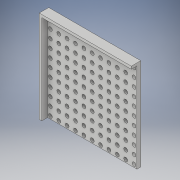
# Autodesk Inventor part: base
Saved by Autodesk Inventor 2018 (Build 220112000, 112)
## iProperties
Created: 2018-04-20
Part Number: base
Material: Generic
Document SubType Name: Modeling
Designer: 4070609
Density: 1 g/cm^3
Appearance: Default
Author: 4070609
Autodesk Inventor part; units mm, degrees
ref_plane "YZ Plane" through (0, 0, 0) normal (1, 0, 0) x (0, 1, 0)
ref_plane "XZ Plane" through (0, 0, 0) normal (0, 1, 0) x (-1, 0, 0)
ref_plane "XY Plane" through (0, 0, 0) normal (0, 0, 1) x (1, 0, 0)
sketch "Sketch1" plane through (0, 0, 0) normal (0, 0, 1) x (1, 0, 0)
  line L0 (0, 0) -> (48.4, 0)
  line L1 (48.4, 0) -> (48.4, 48.4)
  line L2 (48.4, 48.4) -> (0, 48.4)
  line L3 (0, 48.4) -> (0, 0)
  dimension "d0" = 48.4
  dimension "d1" = 48.4
  constraints: 8 end point, 2 parallel, 1 horizontal, 1 perpendicular
  measures "d0" distance of L2.end L1.end
  measures "d1" distance of L1.end L0.end
extrude "Extrusion1" add sketch "Sketch1" along normal blind 2
sketch "Sketch2" plane through (0, 0, 2) normal (0, 0, 1) x (1, 0, 0)
  line L0 (48.4, 0) -> (48.4, 48.4) projected
  line L1 (0, 48.4) -> (0, 0) projected
  line L2 (48.4, 48.4) -> (0, 48.4)
  line L3 (0, 48.4) -> (0, 47)
  line L4 (0, 47) -> (48.4, 47)
  line L5 (48.4, 47) -> (48.4, 48.4)
  line L6 (48.4, 48.4) -> (0, 48.4) projected
  line L7 (0, 0) -> (48.4, 0) projected
  line L8 (0, 48.4) -> (1.4, 48.4)
  line L9 (1.4, 48.4) -> (1.4, 0)
  line L10 (1.4, 0) -> (0, 0)
  line L11 (0, 0) -> (0, 48.4)
  dimension "d4" = 1.4
  dimension "d5" = 1.4
  constraints: 16 end point, 4 parallel, 2 horizontal, 2 perpendicular, 2 point on line
  measures "d4" distance of L3.end L2.end
  measures "d5" distance of L9.end L10.end
extrude "Extrusion2" add sketch "Sketch2" along normal blind 3 contours L4 L9 L2 L0 | L7 L1 L4 L9 | L4 L1 L2 L9
sketch "Sketch3" plane through (0, 0, 2) normal (0, 0, 1) x (1, 0, 0)
  line L0 (48.4, 47) -> (1.4, 47) projected
  line L1 (1.4, 47) -> (2.9, 47)
  line L2 (1.4, 45.5) -> (1.4, 47)
  circle A0 centre (2.9, 45.5) radius 1
  circle A1 centre (7.3, 45.5) radius 1
  circle A2 centre (11.7, 45.5) radius 1
  circle A3 centre (16.1, 45.5) radius 1
  circle A4 centre (20.5, 45.5) radius 1
  circle A5 centre (24.9, 45.5) radius 1
  circle A6 centre (29.3, 45.5) radius 1
  circle A7 centre (33.7, 45.5) radius 1
  circle A8 centre (38.1, 45.5) radius 1
  circle A9 centre (42.5, 45.5) radius 1
  circle A10 centre (46.9, 45.5) radius 1
  line L3 (1.4, 0) -> (1.4, 47) projected
  circle A11 centre (2.9, 41.1) radius 1
  circle A12 centre (7.3, 41.1) radius 1
  circle A13 centre (11.7, 41.1) radius 1
  circle A14 centre (16.1, 41.1) radius 1
  circle A15 centre (20.5, 41.1) radius 1
  circle A16 centre (24.9, 41.1) radius 1
  circle A17 centre (29.3, 41.1) radius 1
  circle A18 centre (33.7, 41.1) radius 1
  circle A19 centre (38.1, 41.1) radius 1
  circle A20 centre (42.5, 41.1) radius 1
  circle A21 centre (46.9, 41.1) radius 1
  circle A22 centre (2.9, 36.7) radius 1
  circle A23 centre (7.3, 36.7) radius 1
  circle A24 centre (11.7, 36.7) radius 1
  circle A25 centre (16.1, 36.7) radius 1
  circle A26 centre (20.5, 36.7) radius 1
  circle A27 centre (24.9, 36.7) radius 1
  circle A28 centre (29.3, 36.7) radius 1
  circle A29 centre (33.7, 36.7) radius 1
  circle A30 centre (38.1, 36.7) radius 1
  circle A31 centre (42.5, 36.7) radius 1
  circle A32 centre (46.9, 36.7) radius 1
  circle A33 centre (2.9, 32.3) radius 1
  circle A34 centre (7.3, 32.3) radius 1
  circle A35 centre (11.7, 32.3) radius 1
  circle A36 centre (16.1, 32.3) radius 1
  circle A37 centre (20.5, 32.3) radius 1
  circle A38 centre (24.9, 32.3) radius 1
  circle A39 centre (29.3, 32.3) radius 1
  circle A40 centre (33.7, 32.3) radius 1
  circle A41 centre (38.1, 32.3) radius 1
  circle A42 centre (42.5, 32.3) radius 1
  circle A43 centre (46.9, 32.3) radius 1
  circle A44 centre (2.9, 27.9) radius 1
  circle A45 centre (7.3, 27.9) radius 1
  circle A46 centre (11.7, 27.9) radius 1
  circle A47 centre (16.1, 27.9) radius 1
  circle A48 centre (20.5, 27.9) radius 1
  circle A49 centre (24.9, 27.9) radius 1
  circle A50 centre (29.3, 27.9) radius 1
  circle A51 centre (33.7, 27.9) radius 1
  circle A52 centre (38.1, 27.9) radius 1
  circle A53 centre (42.5, 27.9) radius 1
  circle A54 centre (46.9, 27.9) radius 1
  circle A55 centre (2.9, 23.5) radius 1
  circle A56 centre (7.3, 23.5) radius 1
  circle A57 centre (11.7, 23.5) radius 1
  circle A58 centre (16.1, 23.5) radius 1
  circle A59 centre (20.5, 23.5) radius 1
  circle A60 centre (24.9, 23.5) radius 1
  circle A61 centre (29.3, 23.5) radius 1
  circle A62 centre (33.7, 23.5) radius 1
  circle A63 centre (38.1, 23.5) radius 1
  circle A64 centre (42.5, 23.5) radius 1
  circle A65 centre (46.9, 23.5) radius 1
  circle A66 centre (2.9, 19.1) radius 1
  circle A67 centre (7.3, 19.1) radius 1
  circle A68 centre (11.7, 19.1) radius 1
  circle A69 centre (16.1, 19.1) radius 1
  circle A70 centre (20.5, 19.1) radius 1
  circle A71 centre (24.9, 19.1) radius 1
  circle A72 centre (29.3, 19.1) radius 1
  circle A73 centre (33.7, 19.1) radius 1
  circle A74 centre (38.1, 19.1) radius 1
  circle A75 centre (42.5, 19.1) radius 1
  circle A76 centre (46.9, 19.1) radius 1
  circle A77 centre (2.9, 14.7) radius 1
  circle A78 centre (7.3, 14.7) radius 1
  circle A79 centre (11.7, 14.7) radius 1
  circle A80 centre (16.1, 14.7) radius 1
  circle A81 centre (20.5, 14.7) radius 1
  circle A82 centre (24.9, 14.7) radius 1
  circle A83 centre (29.3, 14.7) radius 1
  circle A84 centre (33.7, 14.7) radius 1
  circle A85 centre (38.1, 14.7) radius 1
  circle A86 centre (42.5, 14.7) radius 1
  circle A87 centre (46.9, 14.7) radius 1
  circle A88 centre (2.9, 10.3) radius 1
  circle A89 centre (7.3, 10.3) radius 1
  circle A90 centre (11.7, 10.3) radius 1
  circle A91 centre (16.1, 10.3) radius 1
  circle A92 centre (20.5, 10.3) radius 1
  circle A93 centre (24.9, 10.3) radius 1
  circle A94 centre (29.3, 10.3) radius 1
  circle A95 centre (33.7, 10.3) radius 1
  circle A96 centre (38.1, 10.3) radius 1
  circle A97 centre (42.5, 10.3) radius 1
  circle A98 centre (46.9, 10.3) radius 1
  circle A99 centre (2.9, 5.9) radius 1
  circle A100 centre (7.3, 5.9) radius 1
  circle A101 centre (11.7, 5.9) radius 1
  circle A102 centre (16.1, 5.9) radius 1
  circle A103 centre (20.5, 5.9) radius 1
  circle A104 centre (24.9, 5.9) radius 1
  circle A105 centre (29.3, 5.9) radius 1
  circle A106 centre (33.7, 5.9) radius 1
  circle A107 centre (38.1, 5.9) radius 1
  circle A108 centre (42.5, 5.9) radius 1
  circle A109 centre (46.9, 5.9) radius 1
  circle A110 centre (2.9, 1.5) radius 1
  circle A111 centre (7.3, 1.5) radius 1
  circle A112 centre (11.7, 1.5) radius 1
  circle A113 centre (16.1, 1.5) radius 1
  circle A114 centre (20.5, 1.5) radius 1
  circle A115 centre (24.9, 1.5) radius 1
  circle A116 centre (29.3, 1.5) radius 1
  circle A117 centre (33.7, 1.5) radius 1
  circle A118 centre (38.1, 1.5) radius 1
  circle A119 centre (42.5, 1.5) radius 1
  circle A120 centre (46.9, 1.5) radius 1
  point P0 (0, 0)
  dimension "d8" = 1.5
  dimension "d9" = 1.5
  dimension "d10" = 2
  dimension "d13" = 4.4
  dimension "d20" = 4.4
  constraints: 121 centre point, 111 coincident, 4 end point, 2 horizontal, 1 vertical, 350 other
  measures "d8" distance of point (2.9, 45.5) L2.start
  measures "d9" distance of L1.end point (2.9, 45.5)
  measures "d10" diameter of A0
  measures "d13" distance of point (2.9, 45.5) point (7.3, 45.5)
  measures "d20" distance of point (2.9, 45.5) point (2.9, 41.1)
extrude "Extrusion3" cut sketch "Sketch3" against normal blind 3
fillet "Fillet1" radius 0.4 121 edges at (1.9, 45.5, 0) (6.3, 45.5, 0) (10.7, 45.5, 0) (15.1, 45.5, 0) (19.5, 45.5, 0) (23.9, 45.5, 0) (28.3, 45.5, 0) (32.7, 45.5, 0) (37.1, 45.5, 0) (41.5, 45.5, 0) (45.9, 45.5, 0) (45.9, 41.1, 0) (41.5, 41.1, 0) (37.1, 41.1, 0) (32.7, 41.1, 0) (28.3, 41.1, 0) (23.9, 41.1, 0) (19.5, 41.1, 0) (15.1, 41.1, 0) (10.7, 41.1, 0) (6.3, 41.1, 0) (1.9, 41.1, 0) (1.9, 36.7, 0) (6.3, 36.7, 0) (10.7, 36.7, 0) (15.1, 36.7, 0) (19.5, 36.7, 0) (23.9, 36.7, 0) (28.3, 36.7, 0) (32.7, 36.7, 0) (37.1, 36.7, 0) (41.5, 36.7, 0) (45.9, 36.7, 0) (45.9, 32.3, 0) (41.5, 32.3, 0) (37.1, 32.3, 0) (32.7, 32.3, 0) (28.3, 32.3, 0) (23.9, 32.3, 0) (19.5, 32.3, 0) (15.1, 32.3, 0) (10.7, 32.3, 0) (6.3, 32.3, 0) (1.9, 32.3, 0) (1.9, 27.9, 0) (6.3, 27.9, 0) (10.7, 27.9, 0) (15.1, 27.9, 0) (19.5, 27.9, 0) (23.9, 27.9, 0) (28.3, 27.9, 0) (32.7, 27.9, 0) (37.1, 27.9, 0) (41.5, 27.9, 0) (45.9, 27.9, 0) (45.9, 23.5, 0) (41.5, 23.5, 0) (37.1, 23.5, 0) (32.7, 23.5, 0) (28.3, 23.5, 0) (23.9, 23.5, 0) (19.5, 23.5, 0) (15.1, 23.5, 0) (10.7, 23.5, 0) (6.3, 23.5, 0) (1.9, 23.5, 0) (1.9, 19.1, 0) (6.3, 19.1, 0) (10.7, 19.1, 0) (15.1, 19.1, 0) (19.5, 19.1, 0) (23.9, 19.1, 0) (28.3, 19.1, 0) (32.7, 19.1, 0) (37.1, 19.1, 0) (41.5, 19.1, 0) (45.9, 19.1, 0) (45.9, 14.7, 0) (41.5, 14.7, 0) (37.1, 14.7, 0) (32.7, 14.7, 0) (28.3, 14.7, 0) (23.9, 14.7, 0) (19.5, 14.7, 0) (15.1, 14.7, 0) (10.7, 14.7, 0) (6.3, 14.7, 0) (1.9, 14.7, 0) (1.9, 10.3, 0) (6.3, 10.3, 0) (10.7, 10.3, 0) (15.1, 10.3, 0) (19.5, 10.3, 0) (23.9, 10.3, 0) (28.3, 10.3, 0) (32.7, 10.3, 0) (37.1, 10.3, 0) (41.5, 10.3, 0) (45.9, 10.3, 0) (45.9, 5.9, 0) (41.5, 5.9, 0) (37.1, 5.9, 0) (32.7, 5.9, 0) (28.3, 5.9, 0) (23.9, 5.9, 0) (19.5, 5.9, 0) (15.1, 5.9, 0) (10.7, 5.9, 0) (6.3, 5.9, 0) (1.9, 5.9, 0) (1.9, 1.5, 0) (6.3, 1.5, 0) (10.7, 1.5, 0) (15.1, 1.5, 0) (19.5, 1.5, 0) (23.9, 1.5, 0) (28.3, 1.5, 0) (32.7, 1.5, 0) (37.1, 1.5, 0) (41.5, 1.5, 0) (45.9, 1.5, 0)
body "Solid1"
